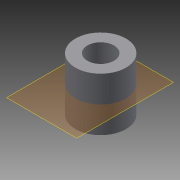
# Autodesk Inventor part: cuscinettoY
Saved by Autodesk Inventor 2014 SP1 (Build 180222100, 222)
## iProperties
Created: 2015-04-08
Part Number: cuscinettoY
Material: Generic
Document SubType Name: Modeling
Designer: Giorgio Nuzzo
Density: 1 g/cm^3
Appearance: Default
d0: 10,000 mm
d1: 20,000 mm
d2: 0,00 deg
Author: Giorgio Nuzzo
Autodesk Inventor part; units mm, degrees
ref_plane "YZ Plane" through (0, 0, 0) normal (1, 0, 0) x (0, 1, 0)
ref_plane "XZ Plane" through (0, 0, 0) normal (0, 1, 0) x (-1, 0, 0)
ref_plane "XY Plane" through (0, 0, 0) normal (0, 0, 1) x (1, 0, 0)
ref_plane "Work Plane1" through (60.2609, 15.8908, 42.5184) normal (0, 0, 1) x (1, 0, 0)
sketch "Sketch1" plane through (60.2609, 15.8908, 42.5184) normal (0, 0, 1) x (1, 0, 0)
  circle A0 centre (0, 1.9992) radius 7.5 projected
  circle A1 centre (0, 1.9992) radius 5
  point P0 (-60.2609, -15.8908)
  dimension "d0" = 10
  constraints: 1 centre point, 1 coincident
  measures "d0" diameter of A1
extrude "Extrusion1" add sketch "Sketch1" along normal mid plane 20
body "Solid1"
